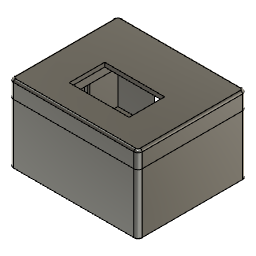
mh-z14a (Autodesk Fusion 360 design; units mm, degrees)
Autodesk Fusion 360 part; units mm, degrees
sketch "Base" plane through (0, 0, 0) normal (0, 0, 1) x (1, 0, 0)
  line L0 (2, 50) -> (59.6, 50)
  line L1 (59.6, 50) -> (59.6, 2)
  line L2 (59.6, 2) -> (2, 2)
  line L3 (2, 2) -> (2, 50)
  line L4 (61.6, 52) -> (61.6, 0)
  line L5 (61.6, 0) -> (0, 0)
  line L6 (0, 0) -> (0, 52)
  line L7 (0, 52) -> (61.6, 52)
  dimension "d1" = 57.6
  dimension "d2" = 48
  dimension "d3" = -2
  constraint horizontal L0
  constraint vertical L1
  constraint horizontal L2
  constraint vertical L3
  constraint coincident L5.end L6.start
  measures "d1" distance of L0.start L0.end
  measures "d2" distance of L0.start L2.end
extrude "Extrude2" add sketch "Base" along normal blind 37 makes body 1
extrude "Extrude1" add sketch "Base" along normal blind 2 separate body contours L0 L1 L2 L3 | L4 L5 L6 L7 makes body 2
sketch "bottom" plane through (0, 0, 2) normal (0, 0, 1) x (-1, 0, 0)
  line L0 (-2, -2) -> (-2, -50)
  line L1 (-2, -50) -> (-59.6, -50)
  line L2 (-59.6, -50) -> (-59.6, -2)
  line L3 (-59.6, -2) -> (-2, -2)
  line L4 (-2, -36) -> (-59.6, -36)
  line L5 (-2, -34) -> (-59.6, -34)
  line L6 (-3.5, -36) -> (-3.5, -34)
  line L7 (-58.1, -36) -> (-58.1, -34)
  line L8 (-2, -2) -> (-54, -2)
  line L9 (-54, -2) -> (-54, -30.7)
  line L10 (-54, -30.7) -> (-2, -30.7)
  line L11 (-2, -30.7) -> (-2, -2)
  line L12 (-56, -2) -> (-56, -32.7)
  line L13 (-56, -32.7) -> (-2, -32.7)
  line L14 (-54, -30.7) -> (-51, -30.7)
  line L15 (-51, -30.7) -> (-51, -27.7)
  line L16 (-51, -27.7) -> (-54, -27.7)
  line L17 (-54, -27.7) -> (-54, -30.7)
  line L18 (-54, -2) -> (-51, -2)
  line L19 (-51, -2) -> (-51, -5)
  line L20 (-51, -5) -> (-54, -5)
  line L21 (-54, -5) -> (-54, -2)
  line L22 (-2, -30.7) -> (-5, -30.7)
  line L23 (-5, -30.7) -> (-5, -27.7)
  line L24 (-5, -27.7) -> (-2, -27.7)
  line L25 (-2, -27.7) -> (-2, -30.7)
  line L26 (-2, -2) -> (-5, -2)
  line L27 (-5, -2) -> (-5, -5)
  line L28 (-5, -5) -> (-2, -5)
  line L29 (-2, -5) -> (-2, -2)
  dimension "d8" = 14
  dimension "d9" = 2
  dimension "d12" = 1.5
  dimension "d13" = 1.5
  dimension "d22" = 52
  dimension "d23" = 28.7
  dimension "d24" = 2
  dimension "d32" = 3
  dimension "d33" = 3
  dimension "d34" = 3
  dimension "d35" = 3
  dimension "d36" = 3
  dimension "d37" = 3
  dimension "d38" = 3
  dimension "d39" = 3
  constraint coincident L0 L4.start
  constraint coincident L2 L4.end
  constraint perpendicular L2 L4
  constraint coincident L0 L5.start
  constraint coincident L2 L5.end
  constraint perpendicular L2 L5
  constraint coincident L4 L6.start
  constraint coincident L5 L6.end
  constraint perpendicular L5 L6
  constraint coincident L4 L7.start
  constraint coincident L5 L7.end
  constraint perpendicular L5 L7
  constraint horizontal L8
  constraint vertical L9
  constraint horizontal L10
  constraint vertical L11
  constraint coincident L0.start L3.end
  constraint horizontal L14
  constraint vertical L15
  constraint horizontal L16
  constraint vertical L17
  constraint horizontal L18
  constraint vertical L19
  constraint horizontal L20
  constraint vertical L21
  constraint horizontal L22
  constraint vertical L23
  constraint horizontal L24
  constraint vertical L25
  constraint horizontal L26
  constraint vertical L27
  constraint horizontal L28
  constraint vertical L29
  measures "d8" distance of L1 L4
  measures "d9" distance of L4 L5
  measures "d12" distance of L0 L6
  measures "d13" distance of L2 L7
  measures "d22" distance of L9.end L10.end
  measures "d23" distance of L8.end L9.end
  measures "d32" distance of L9.end L14.end
  measures "d33" distance of L9.end L16.end
  measures "d34" distance of L8.end L18.end
  measures "d35" distance of L8.end L20.end
  measures "d36" distance of L10.end L22.end
  measures "d37" distance of L10.end L24.end
  measures "d38" distance of L0.start L26.end
  measures "d39" distance of L0.start L28.end
extrude "Extrude4" add sketch "bottom" along normal up to surface (35 mm away) contours L0 L4 L5 L6 | L2 L4 L5 L7 bodies 1 2
extrude "Extrude3" add sketch "bottom" along normal blind 3 contours L0 L4 L5 L6 | L4 L5 L6 L7 | L2 L4 L5 L7 bodies 1
sketch "Window" plane through (0, 50, 0) normal (0, -1, 0) x (1, 0, 0)
  line L0 (2, 2) -> (2, 37)
  line L1 (2, 37) -> (59.6, 37)
  line L2 (59.6, 2) -> (59.6, 37)
  line L3 (2, 2) -> (59.6, 2)
  line L4 (19.5, 25.3) -> (38.9, 25.3)
  line L5 (38.9, 25.3) -> (38.9, 11.3)
  line L6 (38.9, 11.3) -> (19.5, 11.3)
  line L7 (19.5, 11.3) -> (19.5, 25.3)
  line L8 (2, 2) -> (59.6, 2)
  dimension "d16" = 19.4
  dimension "d17" = 14
  dimension "d18" = 9.3
  dimension "d19" = 20.7
  constraint horizontal L4
  constraint vertical L5
  constraint horizontal L6
  constraint vertical L7
  measures "d16" distance of L4.start L4.end
  measures "d17" distance of L4.start L6.end
  measures "d18" distance of L6 L8
  measures "d19" distance of L2 L5
extrude "Extrude5" cut sketch "Window" against normal up to surface (2 mm away) contours L4 L5 L6 L7 bodies 1
extrude "Extrude6" add sketch "bottom" along normal blind 8 contours L0 L3 L9 L10 L12 L13 L14 L17 L21 L22 bodies 1
sketch "microUSB" plane through (2, 0, 0) normal (1, 0, 0) x (0, 1, 0)
  line L0 (30.7, 2) -> (30.7, 10)
  line L1 (30.7, 10) -> (32.7, 10)
  line L2 (32.7, 10) -> (32.7, 2)
  line L3 (32.7, 2) -> (34, 2)
  line L4 (34, 2) -> (34, 37)
  line L5 (34, 37) -> (2, 37)
  line L6 (2, 37) -> (2, 2)
  line L7 (2, 2) -> (30.7, 2)
  line L8 (8, 11) -> (24.7, 11)
  line L9 (24.7, 11) -> (24.7, 2)
  line L10 (24.7, 2) -> (8, 2)
  line L11 (8, 2) -> (8, 11)
  dimension "d27" = 6
  dimension "d28" = 6
  dimension "d29" = 9
  constraint horizontal L8
  constraint vertical L9
  constraint horizontal L10
  constraint vertical L11
  constraint coincident L7 L9.end
  measures "d27" distance of L6 L11
  measures "d28" distance of L0 L9
  measures "d29" distance of L8.start L10.end
extrude "Extrude7" cut sketch "microUSB" against normal up to surface (2 mm away) contours L7 L8 L9 L10 L11 bodies 1
extrude "Extrude8" add sketch "bottom" along normal blind 5 contours L0 L3 L8 L11 L26 L27 L28 L29 | L0 L10 L11 L22 L23 L24 L25 | L3 L8 L9 L18 L19 L20 L21 | L9 L10 L14 L15 L16 L17 bodies 1
extrude "Extrude9" cut 1 faces at (41.0667, 34.6667, 0) along direction (0, 0, 1) blind 1 on bodies 1 bodies 1
fillet "Fillet1" radius 2 4 edges at (0, 0, 19) (61.6, 0, 19) (61.6, 52, 19) (0, 52, 19) on bodies 1
chamfer "Chamfer1" distance 5 distance2 2 4 edges at (38.9, 52, 18.3) (29.2, 52, 25.3) (19.5, 52, 18.3) (29.2, 52, 11.3) measured on face at (52.7, 52, 21.1) measured on face at (52.7, 52, 21.1) measured on face at (52.7, 52, 21.1) measured on face at (52.7, 52, 21.1) on bodies 1
fillet "Fillet2" radius 0.5 8 edges at (0, 26, 1) (0.5858, 0.5858, 1) (30.8, 0, 1) (61.0142, 0.5858, 1) (61.6, 26, 1) (61.0142, 51.4142, 1) (30.8, 52, 1) (0.5858, 51.4142, 1) on bodies 1
sketch "Sketch5" plane through (0, 0, 37) normal (0, 0, 1) x (-1, 0, 0)
  arc A0 (-2, -52) -> (0, -50) centre (-2, -50) ccw
  line L0 (0, -50) -> (0, -2)
  arc A1 (0, -2) -> (-2, 0) centre (-2, -2) ccw
  line L1 (-2, 0) -> (-59.6, 0)
  arc A2 (-59.6, 0) -> (-61.6, -2) centre (-59.6, -2) ccw
  line L2 (-61.6, -2) -> (-61.6, -50)
  arc A3 (-61.6, -50) -> (-59.6, -52) centre (-59.6, -50) ccw
  line L3 (-59.6, -52) -> (-2, -52)
  line L4 (-59.6, -2) -> (-2, -2)
  line L5 (-2, -2) -> (-2, -34)
  line L6 (-2, -34) -> (-3.5, -34)
  line L7 (-3.5, -34) -> (-3.5, -36)
  line L8 (-3.5, -36) -> (-2, -36)
  line L9 (-2, -36) -> (-2, -50)
  line L10 (-2, -50) -> (-59.6, -50)
  line L11 (-59.6, -50) -> (-59.6, -36)
  line L12 (-59.6, -36) -> (-58.1, -36)
  line L13 (-58.1, -36) -> (-58.1, -34)
  line L14 (-58.1, -34) -> (-59.6, -34)
  line L15 (-59.6, -34) -> (-59.6, -2)
  line L16 (-2, -50) -> (-59.6, -50)
  line L17 (-59.6, -50) -> (-59.6, -2)
  line L18 (-59.6, -2) -> (-2, -2)
  line L19 (-2, -2) -> (-2, -50)
  line L20 (-60.4, -50.8) -> (-60.4, -1.2)
  line L21 (-60.4, -1.2) -> (-1.2, -1.2)
  line L22 (-1.2, -1.2) -> (-1.2, -50.8)
  line L23 (-1.2, -50.8) -> (-60.4, -50.8)
  dimension "d50" = -0.8
  constraint horizontal L16
  constraint vertical L17
  constraint horizontal L18
  constraint vertical L19
  constraint coincident A2.centre L4.start
  constraint coincident A0.centre L9.end
extrude "Extrude10" cut sketch "Sketch5" against normal blind 7 contours A0 L0 A1 L1 A2 L2 A3 L3 bodies 1
fillet "Fillet3" radius 1 4 edges at (1.2, 1.2, 33.5) (1.2, 50.8, 33.5) (60.4, 1.2, 33.5) (60.4, 50.8, 33.5) on bodies 1
chamfer "Chamfer2" distance 0.4 angle 45 8 edges at (30.8, 1.2, 37) (60.1071, 1.4929, 37) (60.4, 26, 37) (60.1071, 50.5071, 37) (30.8, 50.8, 37) (1.4929, 50.5071, 37) (1.2, 26, 37) (1.4929, 1.4929, 37) on bodies 1
chamfer "Chamfer3" distance 1 angle 45 1 edges at (58.1, 36, 21) on bodies 1
chamfer "Chamfer4" distance 1 angle 45 1 edges at (3.5, 36, 21) on bodies 1
sketch "Sketch6" plane through (0, 0, 37) normal (0, 0, 1) x (-1, 0, 0)
  arc A0 (-2.2, -50.8) -> (-1.2, -49.8) centre (-2.2, -49.8) ccw
  line L0 (-59.4, -50.8) -> (-2.2, -50.8)
  line L1 (-1.2, -49.8) -> (-1.2, -2.2)
  arc A1 (-60.4, -49.8) -> (-59.4, -50.8) centre (-59.4, -49.8) ccw
  line L2 (-60.4, -2.2) -> (-60.4, -49.8)
  arc A2 (-59.4, -1.2) -> (-60.4, -2.2) centre (-59.4, -2.2) ccw
  line L3 (-2.2, -1.2) -> (-59.4, -1.2)
  arc A3 (-1.2, -2.2) -> (-2.2, -1.2) centre (-2.2, -2.2) ccw
  line L4 (0, -2) -> (0, -50)
  arc A4 (-2, -52) -> (0, -50) centre (-2, -50) ccw
  arc A5 (-61.6, -50) -> (-59.6, -52) centre (-59.6, -50) ccw
  line L5 (-61.6, -50) -> (-61.6, -2)
  arc A6 (-59.6, 0) -> (-61.6, -2) centre (-59.6, -2) ccw
  line L6 (-59.6, 0) -> (-2, 0)
  arc A7 (0, -2) -> (-2, 0) centre (-2, -2) ccw
  line L7 (-2, -52) -> (-59.6, -52)
  line L8 (-59.4, -51) -> (-2.2, -51)
  arc A8 (-2.2, -51) -> (-1, -49.8) centre (-2.2, -49.8) ccw
  line L9 (-1, -49.8) -> (-1, -2.2)
  arc A9 (-1, -2.2) -> (-2.2, -1) centre (-2.2, -2.2) ccw
  line L10 (-2.2, -1) -> (-59.4, -1)
  arc A10 (-59.4, -1) -> (-60.6, -2.2) centre (-59.4, -2.2) ccw
  line L11 (-60.6, -2.2) -> (-60.6, -49.8)
  arc A11 (-60.6, -49.8) -> (-59.4, -51) centre (-59.4, -49.8) ccw
  dimension "d59" = 0.2
  constraint coincident A4.start L7.start
  constraint coincident A5.end L7.end
extrude "Extrude11" add sketch "Sketch6" against normal blind 7 separate body contours L4 A4 A5 L5 A6 L6 A7 L7 makes body 3
sketch "Sketch7" plane through (0, 0, 37) normal (0, 0, 1) x (-1, 0, 0)
  line L0 (-60.6, -2.2) -> (-60.6, -49.8)
  arc A0 (-59.4, -1) -> (-60.6, -2.2) centre (-59.4, -2.2) ccw
  line L1 (-2.2, -1) -> (-59.4, -1)
  arc A1 (-1, -2.2) -> (-2.2, -1) centre (-2.2, -2.2) ccw
  line L2 (-1, -49.8) -> (-1, -2.2)
  arc A2 (-2.2, -51) -> (-1, -49.8) centre (-2.2, -49.8) ccw
  line L3 (-59.4, -51) -> (-2.2, -51)
  arc A3 (-60.6, -49.8) -> (-59.4, -51) centre (-59.4, -49.8) ccw
  line L4 (-59.6, 0) -> (-2, 0)
  arc A4 (-59.6, 0) -> (-61.6, -2) centre (-59.6, -2) ccw
  line L5 (-61.6, -50) -> (-61.6, -2)
  arc A5 (-61.6, -50) -> (-59.6, -52) centre (-59.6, -50) ccw
  line L6 (-2, -52) -> (-59.6, -52)
  arc A6 (-2, -52) -> (0, -50) centre (-2, -50) ccw
  line L7 (0, -2) -> (0, -50)
  arc A7 (0, -2) -> (-2, 0) centre (-2, -2) ccw
  line L8 (-17.45, -28.2) -> (-44.15, -28.2)
  line L9 (-44.15, -28.2) -> (-44.15, -13.2)
  line L10 (-44.15, -13.2) -> (-17.45, -13.2)
  line L11 (-17.45, -13.2) -> (-17.45, -28.2)
  line L12 (-16.9, -4.5) -> (-44.7, -4.5)
  line L13 (-44.7, -4.5) -> (-44.7, -32.7)
  line L14 (-44.7, -32.7) -> (-16.9, -32.7)
  line L15 (-16.9, -32.7) -> (-16.9, -4.5)
  line L16 (-45.7, -3.5) -> (-45.7, -33.7)
  line L17 (-45.7, -33.7) -> (-15.9, -33.7)
  line L18 (-15.9, -33.7) -> (-15.9, -3.5)
  line L19 (-15.9, -3.5) -> (-45.7, -3.5)
  line L20 (-16.9, -4.5) -> (-19.4, -4.5)
  line L21 (-19.4, -4.5) -> (-19.4, -7)
  line L22 (-19.4, -7) -> (-16.9, -7)
  line L23 (-16.9, -7) -> (-16.9, -4.5)
  line L24 (-44.7, -4.5) -> (-42.2, -4.5)
  line L25 (-42.2, -4.5) -> (-42.2, -7)
  line L26 (-42.2, -7) -> (-44.7, -7)
  line L27 (-44.7, -7) -> (-44.7, -4.5)
  line L28 (-44.7, -32.7) -> (-42.2, -32.7)
  line L29 (-42.2, -32.7) -> (-42.2, -30.2)
  line L30 (-42.2, -30.2) -> (-44.7, -30.2)
  line L31 (-44.7, -30.2) -> (-44.7, -32.7)
  line L32 (-16.9, -32.7) -> (-19.4, -32.7)
  line L33 (-19.4, -32.7) -> (-19.4, -30.2)
  line L34 (-19.4, -30.2) -> (-16.9, -30.2)
  line L35 (-16.9, -30.2) -> (-16.9, -32.7)
  dimension "d64" = 26.7
  dimension "d65" = 15
  dimension "d67" = 16.45
  dimension "d71" = 27.8
  dimension "d72" = 28.2
  dimension "d74" = 0.55
  dimension "d76" = 1
  dimension "d79" = 2.5
  dimension "d80" = 2.5
  dimension "d81" = 2.5
  dimension "d82" = 2.5
  dimension "d83" = 2.5
  dimension "d84" = 2.5
  dimension "d85" = 2.5
  dimension "d86" = 2.5
  dimension "d93" = 2.5
  dimension "d94" = 4.5
  constraint horizontal L8
  constraint vertical L9
  constraint horizontal L10
  constraint vertical L11
  constraint horizontal L12
  constraint vertical L13
  constraint horizontal L14
  constraint vertical L15
  constraint horizontal L20
  constraint vertical L21
  constraint horizontal L22
  constraint vertical L23
  constraint horizontal L24
  constraint vertical L25
  constraint horizontal L26
  constraint vertical L27
  constraint horizontal L28
  constraint vertical L29
  constraint horizontal L30
  constraint vertical L31
  constraint horizontal L32
  constraint vertical L33
  constraint horizontal L34
  constraint vertical L35
  measures "d64" distance of L8.start L8.end
  measures "d65" distance of L8.start L10.end
  measures "d67" distance of L2 L11
  measures "d71" distance of L13.end L14.end
  measures "d72" distance of L12.end L13.end
  measures "d74" distance of L9 L13
  measures "d79" distance of L12.start L20.end
  measures "d80" distance of L12.start L22.end
  measures "d81" distance of L12.end L24.end
  measures "d82" distance of L12.end L26.end
  measures "d83" distance of L13.end L28.end
  measures "d84" distance of L13.end L30.end
  measures "d85" distance of L14.end L32.end
  measures "d86" distance of L14.end L34.end
  measures "d93" distance of L1 L19
  measures "d94" distance of L8 L14
extrude "Extrude15" add sketch "Sketch7" against normal blind 1.8 separate body contours L12 L15 L20 L21 L22 L23 | L12 L13 L24 L25 L26 L27 | L14 L15 L32 L33 L34 L35 | L13 L14 L28 L29 L30 L31 makes body 4 at (43.8667, 5.3333, 37) makes body 5 at (43.8667, 31.0333, 37) makes body 6 at (18.5667, 5.3333, 37) makes body 7 at (18.5667, 31.0333, 37)
extrude "Extrude12" add sketch "Sketch7" along normal blind 1 contours L0 A0 L1 A1 L2 A2 L3 A3 | L4 A4 L5 A5 L6 A6 L7 A7 | L8 L9 L10 L11 | L12 L15 L20 L21 L22 L23 | L12 L13 L14 L15 L21 L22 L25 L26 L29 L30 L33 L34 | L12 L13 L24 L25 L26 L27 | L14 L15 L32 L33 L34 L35 | L13 L14 L28 L29 L30 L31 | L16 L17 L18 L19 bodies 3
extrude "Extrude13" cut sketch "Sketch7" along normal up to surface (1 mm away) contours L8 L9 L10 L11 bodies 3
chamfer "Chamfer5" distance 1 angle 45 4 edges at (30.8, 28.2, 38) (44.15, 20.7, 38) (17.45, 20.7, 38) (30.8, 13.2, 38) on bodies 3
extrude "Extrude14" add sketch "Sketch7" against normal blind 4 contours L16 L17 L18 L19 bodies 3
fillet "Fillet4" radius 1 8 edges at (61.0142, 0.5858, 38) (61.6, 26, 38) (61.0142, 51.4142, 38) (30.8, 52, 38) (0.5858, 51.4142, 38) (0, 26, 38) (0.5858, 0.5858, 38) (30.8, 0, 38) on bodies 3
fillet "Fillet5" radius 2 4 edges at (15.9, 3.5, 35) (45.7, 3.5, 35) (45.7, 33.7, 35) (15.9, 33.7, 35) on bodies 3
combine "Combine1" operation add target body 3 tool bodies 4 5 6 7
extrude "Extrude16" add 1 faces at (26.5, 45.2333, 37) along direction (0, 0, -1) blind 0.5 on bodies 3 bodies 3
sketch "Sketch8" plane through (0, 0, 36.5) normal (0, 0, -1) x (1, 0, 0)
named bodies: "bottom", "top"
